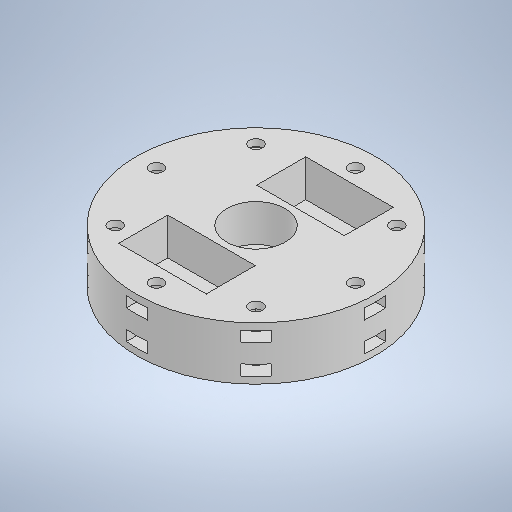
# Autodesk Inventor part: SCARA swivel base - top
Saved by Autodesk Inventor 2025.2 (Build 292293000, 293)
## iProperties
Created: 2025-01-25
Part Number: SCARA swivel base - top
Material: Generic
Document SubType Name: Modeling
Designer: caomi
Density: 1 g/cm^3
Appearance: Default
Author: caomi
Autodesk Inventor part; units mm, degrees
ref_plane "YZ Plane" through (0, 0, 0) normal (1, 0, 0) x (0, 1, 0)
ref_plane "XZ Plane" through (0, 0, 0) normal (0, 1, 0) x (-1, 0, 0)
ref_plane "XY Plane" through (0, 0, 0) normal (0, 0, 1) x (1, 0, 0)
sketch "Sketch1" plane through (0, 0, 0) normal (0, 1, 0) x (-1, 0, 0)
  circle A0 centre (0, 0) radius 45
  line L0 (20, 13.25) -> (-13, 13.25)
  line L1 (-13, 13.25) -> (-13, 31.75)
  line L2 (-13, 31.75) -> (20, 31.75)
  line L3 (45.5655, 22.5) -> (-15.5039, 22.5) construction
  line L4 (0, -63) -> (0, 63) projected
  line L5 (-20, -31.75) -> (13, -31.75)
  line L6 (13, -31.75) -> (13, -13.25)
  line L7 (13, -13.25) -> (-20, -13.25)
  line L8 (19.1191, -22.5) -> (-71.9329, -22.5) construction
  line L9 (69.0652, 0) -> (-95.4326, 0) projected
  circle A1 centre (0, 0) radius 11
  circle A2 centre (0, 0) radius 4
  line L10 (20, 13.25) -> (20, 31.75)
  line L11 (-20, -13.25) -> (-20, -31.75)
  circle A3 centre (13, 22.5) radius 1.6
  circle A4 centre (-13, -22.5) radius 1.6
  line L12 (10, 20.7679) -> (10, 24.2321)
  line L13 (10, 24.2321) -> (13, 25.9641)
  line L14 (13, 25.9641) -> (16, 24.2321)
  line L15 (16, 24.2321) -> (16, 20.7679)
  line L16 (16, 20.7679) -> (13, 19.0359)
  line L17 (13, 19.0359) -> (10, 20.7679)
  line L18 (-13, -25.9641) -> (-16, -24.2321)
  line L19 (-16, -24.2321) -> (-16, -20.7679)
  line L20 (-16, -20.7679) -> (-13, -19.0359)
  line L21 (-13, -19.0359) -> (-10, -20.7679)
  line L22 (-10, -20.7679) -> (-10, -24.2321)
  line L23 (-10, -24.2321) -> (-13, -25.9641)
  point P0 (0, -4.3524)
  point P1 (0, -22.5)
  point P2 (0, 22.5)
  point P3 (0, 22.5)
  point P4 (0, -22.5)
  dimension "d1" = 18.5
  dimension "d2" = 90
  dimension "d12" = 22
  dimension "d26" = 45
  dimension "d50" = 8
  dimension "d53" = 33
  dimension "d54" = 20
  dimension "d55" = 20
  dimension "d56" = 3.2
  dimension "d57" = 7
  dimension "d59" = 7
  dimension "d60" = 6
  dimension "d61" = 6
  constraints: 44 end point, 7 point on line, 5 centre point, 4 coincident, 4 vertical, 3 horizontal, 3 perpendicular, 3 vertical alignment, 2 parallel, 1 equal radius, 1 midpoint, 30 other
  measures "d1" distance of L0.end L1.end
  measures "d2" diameter of A0
  measures "d12" diameter of A1
  measures "d26" distance of point (0, 22.5) point (0, -22.5)
  measures "d50" diameter of A2
  measures "d53" distance of L1.end L2.end
  measures "d54" distance from line of L10 point (0, 22.5)
  measures "d55" distance from line of L11 point (0, -22.5)
  measures "d56" diameter of A3
  measures "d57" distance from line of L10 A3.centre
  measures "d59" distance from line of L11 A4.centre
  measures "d60" distance between parallel lines of L12 L15
  measures "d61" distance between parallel lines of L22 L19
extrude "Extrusion1" add sketch "Sketch1" along normal blind 20 contours L9 A1 L4 L0 L10 L2 A0 | A0 L4 L5 L6 L7 A1 L9 | L4 L2 L1 L0 A1 L9 A0 | A0 L9 A1 L4 L7 L11 L5 | L4 L0 L1 L2 | L2 L10 L0 L4 | L5 L11 L7 L4 | L4 L7 L6 L5 | A3 | A4 | L12 L13 L14 L15 L16 L17 | L18 L19 L20 L21 L22 L23
extrude "Extrusion2" cut sketch "Sketch1" against normal blind 14 from surface at 20 contours L4 L0 L1 L2 | L2 L10 L0 L4 | L5 L11 L7 L4 | L4 L7 L6 L5 | A3 | A4 | L12 L13 L14 L15 L16 L17 | L18 L19 L20 L21 L22 L23
extrude "Extrusion9" cut sketch "Sketch1" along normal blind 5 contours A3 | A4 | L12 L13 L14 L15 L16 L17 | L18 L19 L20 L21 L22 L23
extrude "Extrusion10" cut sketch "Sketch1" along normal up to surface (6 mm away) contours A3 | A4
extrude "Extrusion6" add sketch "Sketch1" along normal up to surface (6 mm away) contours A1 L4 A2 L9 | L9 A2 L4 A1 | A2 L4 L9 | L9 L4 A2 | L4 A2 L9 A1 | A1 L9 A2 L4 | L9 A2 L4 | L4 A2 L9
sketch "Sketch4" plane through (0, 20, 0) normal (0, 1, 0) x (1, 0, 0)
  circle A0 centre (-37.5, 0) radius 2.5
  line L0 (-52.889, 4) -> (-35.4144, 4)
  line L1 (-35.4144, 4) -> (-33.105, 0)
  line L2 (-33.105, 0) -> (-35.4144, -4)
  line L3 (-35.4144, -4) -> (-52.889, -4)
  line L4 (-52.889, -4) -> (-52.889, 4)
  line L5 (0, 0) -> (-69.9236, 0) construction
  circle A1 centre (0, 0) radius 45 projected
  dimension "d32" = 5
  dimension "d33" = 60
  dimension "d34" = 8
  dimension "d35" = 4.395
  dimension "d44" = 37.5
  constraints: 12 end point, 2 horizontal, 1 centre point, 1 parallel, 1 point on line, 1 vertical, 2 other
  measures "d32" diameter of A0
  measures "d33" angle of L1 L5
  measures "d34" distance between parallel lines of L0 L3
  measures "d35" distance of L1.end A0.centre
  measures "d44" distance of A0.centre A1.centre
ref_plane "Work Plane2" through (0, 15.5, 0) normal (0, 1, 0) x (1, 0, 0)
ref_plane "Work Plane3" through (0, 4.5, 0) normal (0, 1, 0) x (1, 0, 0)
extrude "Extrusion4" cut sketch "Sketch4" along normal mid plane 4 from surface at -15.5 contours A0 | L0 A1 L3 L4 | L0 L1 L2 L3 A1 picked at (-39.5409, -3.4458)
extrude "Extrusion5" cut sketch "Sketch4" along normal mid plane 4 from surface at -4.5 contours A0 | L0 A1 L3 L4 | L0 L1 L2 L3 A1 picked at (-39.5409, -3.4458)
extrude "Extrusion7" cut sketch "Sketch4" against normal up to surface (20 mm away) contours A0
pattern_circular "Circular Pattern1" count 8 over 360 about axis through (0, 0, 0) along (0, 1, 0) of "Extrusion5", "Extrusion4", "Extrusion7"
body "Solid1"
